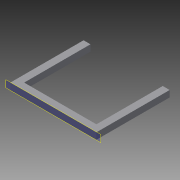
# Autodesk Inventor part: rail
Saved by Autodesk Inventor 2015 (Build 190159000, 159)
## iProperties
Created: 2015-10-18
Part Number: rail
Material: 一般
Document SubType Name: Modeling
Designer: omae
Density: 1 g/cm^3
Appearance: 既定
Author: omae
Autodesk Inventor part; units mm, degrees
ref_plane "YZ Plane" through (0, 0, 0) normal (1, 0, 0) x (0, 1, 0)
ref_plane "XY Plane" through (0, 0, 0) normal (0, 0, 1) x (1, 0, 0)
sketch "スケッチ2" plane through (0, 0, 0) normal (0, 0, 1) x (1, 0, 0)
  line L0 (2279, 0) -> (2279, 1939)
  line L1 (0, 1939.0001) -> (183.5291, 1939.0001)
  line L2 (183.5291, 1939.0001) -> (183.5291, 183.5291)
  line L3 (183.5291, 0) -> (0, 0)
  line L4 (0, 0) -> (0, 1939.0001)
  line L5 (0, 0) -> (2279, 0)
  line L6 (2279, 0) -> (2279, 183.5291)
  line L7 (2095.4709, 183.5291) -> (183.5291, 183.5291)
  line L8 (0, 183.5291) -> (0, 0)
  line L9 (2279, 0) -> (2095.4709, 0)
  line L10 (2095.4709, 183.5291) -> (2095.4709, 1939)
  line L11 (2095.4709, 1939) -> (2279, 1939)
  line L12 (2279, 1939) -> (2279, 0)
  line L13 (2279, 1939) -> (2095.4709, 1939)
  line L14 (183.5291, 1939.0001) -> (0, 1939.0001)
  dimension "d10" = 2279
  dimension "d11" = 1939
  dimension "d12" = 1755.4709
  dimension "d13" = 1755.471
  constraints: 30 end point, 6 parallel, 3 horizontal, 3 perpendicular
  measures "d10" distance between parallel lines of L4 L0
  measures "d11" distance between parallel lines of L11 L5
  measures "d12" distance between parallel lines of L11 L7
  measures "d13" distance between parallel lines of L1 L7
extrude "押し出し1" add sketch "スケッチ2" along normal blind 170
